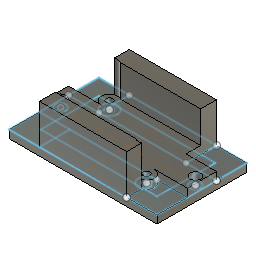
LM2596 Mount (Autodesk Fusion 360 design; units mm, degrees)
Autodesk Fusion 360 part; units mm, degrees
note: some values were not read from the file. Set by a fixed rule: which face or edge a step refers to.
sketch "Sketch1" plane through (0, 0, 0) normal (0, 0, 1) x (1, 0, 0) in component "base"
  line L0 (-13.6644, 20.5385) -> (30.3356, 20.5385)
  line L1 (30.3356, 20.5385) -> (30.3356, -1.4615)
  line L2 (30.3356, -1.4615) -> (-13.6644, -1.4615)
  line L3 (-13.6644, -1.4615) -> (-13.6644, 20.5385)
  line L4 (36.3356, -7.4615) -> (-19.6644, -7.4615)
  line L5 (-19.6644, -7.4615) -> (-19.6644, 26.5385)
  line L6 (-19.6644, 26.5385) -> (36.3356, 26.5385)
  line L7 (36.3356, 26.5385) -> (36.3356, -7.4615)
  line L8 (-13.6644, 9.5385) -> (30.3356, 9.5385) construction
  line L9 (-19.6644, 4.0385) -> (36.3356, 4.0385)
  line L10 (-19.6644, 15.0385) -> (36.3356, 15.0385)
  line L11 (8.3356, 26.5385) -> (8.3356, -7.4615) construction
  line L12 (-8.1644, 4.0385) -> (-8.1644, -7.4615)
  line L13 (24.8356, 4.0385) -> (24.8356, -7.4615)
  line L14 (-8.1644, 15.0385) -> (-8.1644, 26.5385)
  line L15 (24.8356, 15.0385) -> (24.8356, 26.5385)
  circle A0 centre (-17.1644, 9.5385) radius 1
  circle A1 centre (-17.1644, 9.5385) radius 2
  circle A2 centre (33.8356, 9.5385) radius 2
  circle A3 centre (33.8356, 9.5385) radius 1
  circle A4 centre (-7.1644, 18.0385) radius 1.25
  circle A5 centre (23.8356, 1.0385) radius 1.25
  circle A6 centre (-7.1644, 18.0385) radius 3
  circle A7 centre (23.8356, 1.0385) radius 3
  dimension "d1" = 44
  dimension "d2" = 22
  dimension "d3" = -6
  dimension "d7" = 5.5
  dimension "d16" = 5.5
  dimension "d17" = 2
  dimension "d18" = 4
  dimension "d19" = 25.5
  dimension "d20" = 56
  dimension "d27" = 2.5
  dimension "d28" = 2.5
  dimension "d29" = 15.5
  dimension "d30" = 15.5
  dimension "d37" = 6
  dimension "d38" = 6
  dimension "d42" = 2.5
  dimension "d43" = 2.5
  constraint horizontal L0
  constraint vertical L1
  constraint horizontal L2
  constraint vertical L3
  constraint midpoint L3 L8.start
  constraint midpoint L1 L8.end
  constraint coincident L5 L9.start
  constraint coincident L7 L9.end
  constraint perpendicular L7 L9
  constraint symmetric L8 L9.start L10.start
  constraint symmetric L8 L9.end L10.end
  constraint midpoint L6 L11.start
  constraint midpoint L4 L11.end
  constraint coincident L9 L12.start
  constraint coincident L4 L12.end
  constraint perpendicular L4 L12
  constraint symmetric L11 L12.start L13.start
  constraint symmetric L11 L12.end L13.end
  constraint symmetric L8 L12.start L14.start
  constraint symmetric L8 L12.end L14.end
  constraint symmetric L8 L13.start L15.start
  constraint symmetric L8 L13.end L15.end
  constraint coincident L8 A0.centre
  constraint concentric A0 A1
  constraint symmetric L11 A0 A3
  constraint symmetric L11 A1 A2
  constraint concentric A4 A6
  constraint concentric A5 A7
  measures "d1" distance of L0.start L0.end
  measures "d2" distance of L0.start L2.end
  measures "d7" distance of L8 L9
  measures "d16" distance of L3 L12
  measures "d17" diameter of A0
  measures "d18" diameter of A1
  measures "d19" distance of L11 A0.centre
  measures "d20" distance of L5 L7
  measures "d27" diameter of A4
  measures "d28" diameter of A5
  measures "d29" distance of L11 A5.centre
  measures "d30" distance of L11 A4.centre
  measures "d37" diameter of A6
  measures "d38" diameter of A7
  measures "d42" distance of L0 A4.centre
  measures "d43" distance of L2 A5.centre
extrude "Extrude1" add sketch "Sketch1" against normal blind 3 contours L0 L3 L5 L6 L10 L14 A6 | L0 L3 L10 L14 A6 | L0 L14 A6 | L0 L14 A4 A6 | L1 L3 L9 L10 | L3 L5 L9 L10 | L0 L14 A6 | L0 L14 A4 A6 | L0 L6 L14 L15 A6 | L10 L14 A6 | L2 L3 L9 L12 | L2 L3 L4 L5 L9 L12 | L0 L10 L15 A6 | L14 A4 | L14 A4 | L2 L9 L12 A7 | L0 L1 L6 L7 L10 L15 | L0 L1 L10 L15 | L2 L4 L12 L13 A7 | L9 L13 A7 | L2 L13 A5 A7 | L1 L7 L9 L10 | L2 L13 A7 | L1 L2 L9 L13 A7 | L2 L13 A5 A7 | L1 L2 L4 L7 L9 L13 A7 | L2 L13 A7 | L13 A5 | L13 A5 | A0 | A1 | A2 | A3 in component "base"
extrude "Extrude3" add sketch "Sketch1" along normal blind 3 contours L0 L14 A6 | L0 L14 A4 A6 | L1 L3 L9 L10 | L3 L5 L9 L10 | L0 L14 A6 | L0 L14 A4 A6 | L0 L6 L14 L15 A6 | L0 L10 L15 A6 | L14 A4 | L14 A4 | L2 L9 L12 A7 | L2 L4 L12 L13 A7 | L2 L13 A5 A7 | L1 L7 L9 L10 | L2 L13 A7 | L2 L13 A5 A7 | L2 L13 A7 | L13 A5 | L13 A5 in component "base"
extrude "Extrude4" add sketch "Sketch1" along normal blind 15 contours L0 L14 A6 | L0 L6 L14 L15 A6 | L2 L4 L12 L13 A7 | L2 L13 A7 picked at (-6.5068, 20.6041) picked at (23.1781, -1.5271) in component "base"
extrude "Extrude5" cut sketch "Sketch1" along normal up to surface (15 mm away) contours A0 | A1 | A2 | A3 in component "base"
extrude "Extrude6" cut sketch "Sketch1" against normal blind 1.5 contours A1 | A2 in component "base"
extrude "Extrude7" cut sketch "Sketch1" against normal up to surface (3 mm away) contours A0 | A3 in component "base"
extrude "Extrude8" cut sketch "Sketch1" along normal up to surface (3 mm away) and the other way up to surface (3 mm away) contours L14 A4 | L14 A4 | L13 A5 | L13 A5 in component "base"
extrude "Extrude9" cut sketch "Sketch1" along normal up to surface (12 mm away) from surface at 3 contours L0 L14 A6 | L0 L14 A4 A6 | L0 L14 A6 | L0 L14 A4 A6 | L2 L13 A5 A7 | L2 L13 A7 | L2 L13 A5 A7 | L2 L13 A7 in component "base"
component "base" placed x (1, 0, 0) y (0, 1, 0) z (0, 0, 1) at (0, 0, 0)
equation "d19 = ( 51 / 2 ) * 1 mm"
equation "d29 = ( 31 / 2 ) * 1 mm"
equation "d30 = ( 31 / 2 ) * 1 mm"
